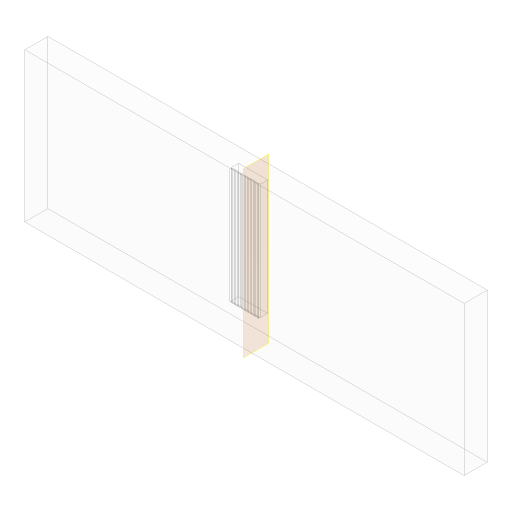
# Autodesk Inventor part: 00_chipnano_waveguide_slidsize_modified
Saved by Autodesk Inventor 2024.1 (Build 281209000, 209)
## iProperties
Created: 2021-12-30
Part Number: 00_chipnano_waveguide_slidsize_modified
Material: Generisch
Document SubType Name: Modeling
Designer: diederichbenedict
Density: 1 g/cm^3
Appearance: Polycarbonat - klar
Author: diederichbenedict
Autodesk Inventor part; units mm, degrees
ref_plane "YZ Plane" through (0, 0, 0) normal (1, 0, 0) x (0, 1, 0)
ref_plane "XZ Plane" through (0, 0, 0) normal (0, 1, 0) x (-1, 0, 0)
ref_plane "XY Plane" through (0, 0, 0) normal (0, 0, 1) x (1, 0, 0)
sketch "Skizze1" plane through (0, 0, 0) normal (0, 0, 1) x (1, 0, 0)
  line L0 (38, -12.9) -> (-38, -12.9)
  line L1 (-38, -12.9) -> (-38, 12.9)
  line L2 (-38, 12.9) -> (38, 12.9)
  line L3 (38, 12.9) -> (38, -12.9)
  line L4 (38, -12.9) -> (-38, 12.9) construction
  line L5 (-38, -12.9) -> (38, 12.9) construction
  point P0 (0, 0)
  dimension "d0" = 76
  dimension "d1" = 25.8
  constraints: 12 end point, 2 midpoint, 2 parallel, 1 horizontal, 1 perpendicular
  measures "d0" distance of L1.end L2.end
  measures "d1" distance of L0.end L1.end
extrude "Extrusion1" add sketch "Skizze1" along normal blind 4
sketch "Skizze2" plane through (0, 0, 4) normal (0, 0, 1) x (1, 0, 0)
  line L0 (38, 12.9) -> (-38, 12.9) projected
  line L1 (-38, 12.9) -> (-38, -12.9) projected
  line L2 (-38, -12.9) -> (38, -12.9) projected
  line L3 (38, -12.9) -> (38, 12.9) projected
  line L4 (2.5, -7.1) -> (-2.5, -7.1)
  line L5 (-2.5, -7.1) -> (-2.5, 12.9)
  line L6 (-2.5, 12.9) -> (2.5, 12.9)
  line L7 (2.5, 12.9) -> (2.5, -7.1)
  line L8 (2.5, -7.1) -> (-2.5, 12.9) construction
  line L9 (-2.5, -7.1) -> (2.5, 12.9) construction
  point P0 (0, 0)
  point P1 (0, 2.9)
  point P2 (0, 12.9)
  dimension "d4" = 5
  dimension "d5" = 20
  constraints: 12 end point, 4 midpoint, 2 parallel, 1 horizontal, 1 perpendicular
  measures "d4" distance of L5.end L6.end
  measures "d5" distance of L4.end L5.end
extrude "Extrusion2" cut sketch "Skizze2" against normal blind 1.5 contours L7 L4 L5 L0
sketch "Skizze3" plane through (-38, 12.9, 0) normal (0, 1, 0) x (1, 0, 0)
  line L0 (40.5, -4) -> (35.5, -4) projected
  line L1 (40.5, -4) -> (40.5, -2.5) projected
  line L2 (40.5, -2.5) -> (35.5, -2.5) projected
  line L3 (35.5, -4) -> (35.5, -2.5) projected
  circle A0 centre (38, -3.875) radius 0.125
  point P0 (38, 0)
  dimension "d8" = 0.25
  constraints: 1 centre point, 1 tangent
  measures "d8" diameter of A0
extrude "Extrusion3" add sketch "Skizze3" against normal up to surface (20 mm away) contours A0
pattern_linear "Rechteckige Anordnung1" count 11 spacing 0.25 along (-1, 0, 0) count 11 spacing 0.25 along (1, 0, 0) of "Extrusion3"
ref_plane "Arbeitsebene1" through (0, -12.9, 0) normal (1, 0, 0) x (0, 0, -1)
